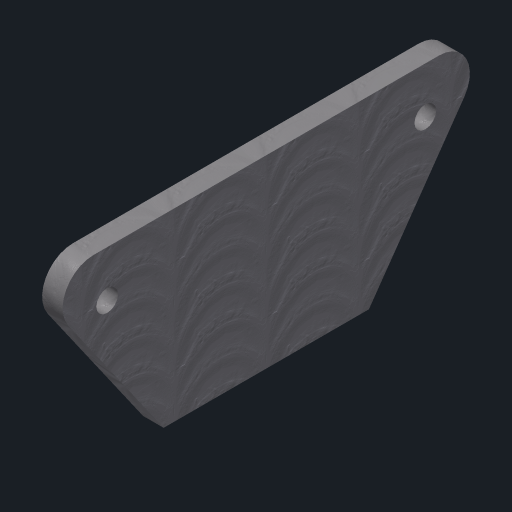
# Autodesk Inventor part: CAJA
Saved by Autodesk Inventor 2024.3 (Build 283343000, 343)
## iProperties
Created: 2024-06-29
Part Number: CAJA
Material: Steel, Mild, Welded
Document SubType Name: Modeling
Designer: Niler
Density: 7.85 g/cm^3
Appearance: Weld - Steel Mild
Author: Niler
Autodesk Inventor part; units mm, degrees
ref_plane "YZ Plane" through (0, 0, 0) normal (1, 0, 0) x (0, 1, 0)
ref_plane "XZ Plane" through (0, 0, 0) normal (0, 1, 0) x (-1, 0, 0)
ref_plane "XY Plane" through (0, 0, 0) normal (0, 0, 1) x (1, 0, 0)
sketch "Sketch1" plane through (0, 0, 0) normal (1, 0, 0) x (0, 1, 0)
  line L0 (-67.5, 145) -> (67.5, 145)
  line L1 (67.5, 145) -> (67.5, -145)
  line L2 (67.5, -145) -> (-67.5, -145)
  line L3 (-67.5, -145) -> (-67.5, 145)
  line L4 (-67.5, 145) -> (67.5, -145) construction
  line L5 (67.5, 145) -> (-67.5, -145) construction
  circle A0 centre (0, 77.5) radius 5.3
  circle A1 centre (0, -77.5) radius 5.3
  circle A2 centre (0, 0) radius 5.3
  line L6 (0, 77.5) -> (0, -77.5) construction
  line L7 (57.5, -135) -> (57.5, 135)
  line L8 (57.5, 135) -> (-57.5, 135)
  line L9 (-57.5, 135) -> (-57.5, -135)
  line L10 (-57.5, -135) -> (57.5, -135)
  dimension "d0" = 155
  dimension "d1" = 10.6
  dimension "d2" = 290
  dimension "d3" = 135
  dimension "d4" = 10
  constraints: 22 end point, 4 parallel, 3 centre point, 3 midpoint, 2 equal radius, 2 perpendicular, 2 vertical alignment, 1 coincident, 1 horizontal, 1 vertical, 3 other
  measures "d0" distance of L6.end L6.start
  measures "d1" diameter of A0
  measures "d2" distance between parallel lines of L2 L0
  measures "d3" distance of L0.start L0.end
  measures "d4" distance between parallel lines of L1 L7
extrude "Extrusion1" add sketch "Sketch1" along normal blind 10 contours L0 L1 L2 L3 | A2 | L10 L9 L8 L7
chamfer "Chamfer2" distance 20 angle 45 4 edges at (5, 67.5, -145) (5, -67.5, -145) (5, -67.5, 145) (5, 67.5, 145)
sketch "Sketch5" plane through (10, 0, 0) normal (1, 0, 0) x (0, 0, -1)
  line L0 (50, -67.5) -> (-50, -67.5) projected
  circle A0 centre (0, -15) radius 11 projected
  circle A1 centre (33.234, -33.234) radius 2.75 projected
  circle A2 centre (-33.234, -33.234) radius 2.75 projected
  line L1 (96.4912, -1.1036) -> (50, -67.5) projected
  line L2 (-50, -67.5) -> (-96.4912, -1.1036) projected
  arc A3 (-84.2039, 22.5) -> (-96.4912, -1.1036) centre (-84.2039, 7.5) ccw projected
  line L3 (-84.2039, 22.5) -> (84.2039, 22.5) projected
  arc A4 (96.4912, -1.1036) -> (84.2039, 22.5) centre (84.2039, 7.5) ccw projected
  circle A5 centre (-18.3535, 19) radius 1.5 projected
  circle A6 centre (18.3535, -64) radius 1.5 projected
  circle A7 centre (18.3535, 19) radius 1.5 projected
  circle A8 centre (-18.3535, -64) radius 1.5 projected
  point P0 (0, 0)
extrude "Extrusion4" [suppressed]
sketch "Sketch6" plane through (10, 0, 0) normal (1, 0, 0) x (0, 0, -1)
  line L0 (-145, 47.5) -> (-125, 67.5) projected
  line L1 (-145, 47.5) -> (-145, -47.5) projected
  line L2 (-125, -67.5) -> (-145, -47.5) projected
  line L3 (-125, -67.5) -> (125, -67.5) projected
  line L4 (145, -47.5) -> (125, -67.5) projected
  line L5 (145, -47.5) -> (145, 47.5) projected
  line L6 (125, 67.5) -> (145, 47.5) projected
  line L7 (125, 67.5) -> (-125, 67.5) projected
  circle A0 centre (-77.5, 0) radius 5.3 projected
  circle A1 centre (77.5, 0) radius 5.3 projected
  circle A2 centre (-131.5, 54) radius 2.9
  circle A3 centre (-96.5, -41.5) radius 2.9
  circle A4 centre (96.5, -41.5) radius 2.9
  circle A5 centre (111.5, 46.5) radius 2.9
  point P0 (0, 0)
  dimension "d21" = 5.8
  constraints: 4 centre point, 3 equal radius
  measures "d21" diameter of A2
extrude "Extrusion5" cut sketch "Sketch6" against normal blind 3.5 contours A2 | A3 | A4 | A5
fillet "Fillet1" radius 5 2 edges at (0, -5.3, 77.5) (0, -5.3, -77.5)
sketch "Sketch7" plane through (10, 0, 0) normal (1, 0, 0) x (0, 0, -1)
  circle A0 centre (96.5, -41.5) radius 2.9 projected
  circle A1 centre (-96.5, -41.5) radius 2.9 projected
  circle A2 centre (111.5, 46.5) radius 2.9 projected
  circle A3 centre (-131.5, 54) radius 2.9 projected
  line L0 (-145, 47.5) -> (-125, 67.5) projected
  line L1 (-145, 47.5) -> (-145, -47.5) projected
  line L2 (-125, -67.5) -> (-145, -47.5) projected
  line L3 (-125, -67.5) -> (125, -67.5) projected
  line L4 (145, -47.5) -> (125, -67.5) projected
  line L5 (145, -47.5) -> (145, 47.5) projected
  line L6 (125, 67.5) -> (145, 47.5) projected
  line L7 (125, 67.5) -> (-125, 67.5) projected
  circle A4 centre (-77.5, 0) radius 5.3 projected
  circle A5 centre (77.5, 0) radius 5.3 projected
  line L8 (0, -67.5) -> (0, 22.5)
  line L9 (0, 22.5) -> (-84.2039, 22.5)
  line L10 (-96.4912, -1.1036) -> (-50, -67.5)
  line L11 (-125, -67.5) -> (125, -67.5) projected
  arc A6 (-84.2039, 22.5) -> (-96.4912, -1.1036) centre (-84.2039, 7.5) ccw
  line L12 (0, 22.5) -> (84.2039, 22.5)
  line L13 (96.4912, -1.1036) -> (50, -67.5)
  arc A7 (96.4912, -1.1036) -> (84.2039, 22.5) centre (84.2039, 7.5) ccw
  point P0 (0, 0)
  point P1 (-50, -67.5)
  point P2 (50, -67.5)
  dimension "d27" = 90
  dimension "d28" = 15
  dimension "d29" = 50
  dimension "d30" = 55
  constraints: 10 end point, 4 point on circle, 4 symmetric about line, 2 centre point, 2 midpoint, 2 tangent, 1 perpendicular, 1 point on line, 1 vertical, 1 other
  measures "d27" distance of L8.start L8.end
  measures "d28" radius of A6
  measures "d29" distance of point (0, -67.5) L10.end
  measures "d30" angle of L11 L10
extrude "Extrusion6" cut sketch "Sketch7" against normal through all contours A0 | A1 | A2 | A3 | L0 L7 L6 L5 L4 L3 L13 A7 L12 L9 A6 L10 L2 L1
body "Solid1"
